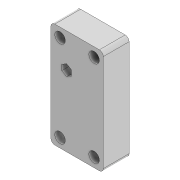
# Autodesk Inventor part: 10_Mountinplate_Mirrors_v2_Special_Combiner
Saved by Autodesk Inventor 2022 (Build 260153000, 153)
## iProperties
Created: 2022-05-18
Part Number: 10_Mountinplate_Mirrors_v2_Special_Combiner
Material: Generisch
Document SubType Name: Modeling
Designer: diederichbenedict
Density: 1 g/cm^3
Appearance: Vorgabe
Author: diederichbenedict
Autodesk Inventor part; units mm, degrees
ref_plane "YZ Plane" through (0, 0, 0) normal (1, 0, 0) x (0, 1, 0)
ref_plane "XZ Plane" through (0, 0, 0) normal (0, 1, 0) x (-1, 0, 0)
ref_plane "XY Plane" through (0, 0, 0) normal (0, 0, 1) x (1, 0, 0)
ref_plane "Arbeitsebene1" through (0.0075, -0.0423, 0) normal (0, 0, 1) x (1, 0, 0)
sketch "Skizze1" plane through (0.0075, -0.0423, 0) normal (0, 0, 1) x (1, 0, 0)
  line L0 (0.635, 25.527) -> (10.16, 25.527) projected
  line L1 (0.635, 25.527) -> (0.635, 0) projected
  line L2 (0.635, 0) -> (10.16, 0) projected
  line L3 (10.16, 0) -> (10.16, 25.527) projected
  line L4 (30.08, -27.3) -> (-3.92, -27.3)
  line L5 (-6.92, -24.3) -> (-6.92, 49.7)
  line L6 (-3.92, 52.7) -> (30.08, 52.7)
  line L7 (33.08, -27.3) -> (-6.92, 52.7) construction
  line L8 (-6.92, -27.3) -> (33.08, 52.7) construction
  arc A0 (30.08, -27.3) -> (33.08, -24.3) centre (30.08, -24.3) ccw
  arc A1 (-6.92, -24.3) -> (-3.92, -27.3) centre (-3.92, -24.3) ccw
  arc A2 (-3.92, 52.7) -> (-6.92, 49.7) centre (-3.92, 49.7) ccw
  arc A3 (33.08, 49.7) -> (30.08, 52.7) centre (30.08, 49.7) ccw
  circle A4 centre (5.08, 12.7) radius 2.3813
  line L9 (33.08, -24.3) -> (33.08, 49.7)
  line L10 (5.08, 12.7) -> (5.08, 26.7)
  circle A5 centre (5.08, 26.7) radius 2.3813
  point P0 (-0.0075, 0.0423)
  point P1 (13.08, 12.7)
  dimension "d1" = 80
  dimension "d2" = 3
  dimension "d7" = 0
  dimension "d8" = 8
  dimension "d37" = 14
  constraints: 14 end point, 8 point on circle, 7 tangent, 6 centre point, 6 point on line, 3 equal radius, 2 vertical, 1 horizontal, 1 midpoint, 1 parallel, 1 perpendicular, 2 other
  measures "d1" distance of L8.start L7.end
  measures "d2" radius of A0
  measures "d7" vertical distance of L10.start point (13.08, 12.7)
  measures "d8" distance of point (13.08, 12.7) L10.start
  measures "d37" distance of L10.start L10.end
ref_plane "Arbeitsebene2" through (291.5074, -13.3966, 8.6065) normal (0, 0, 1) x (0.898794, -0.4383711, 0)
extrude "Extrusion1" add sketch "Skizze1" along normal blind 18.412 contours L0 A5 L3 L2 L1 | L4 A1 L5 A2 L6 A3 L9 A0 | A4
sketch "Skizze3" plane through (0.0075, -0.0423, 0) normal (0, 0, -1) x (-1, 0, 0)
  arc A0 (-30.08, 52.7) -> (-33.08, 49.7) centre (-30.08, 49.7) ccw projected
  line L0 (-33.08, -24.3) -> (-33.08, 49.7) projected
  arc A1 (-33.08, -24.3) -> (-30.08, -27.3) centre (-30.08, -24.3) ccw projected
  line L1 (3.92, -27.3) -> (-30.08, -27.3) projected
  arc A2 (3.92, -27.3) -> (6.92, -24.3) centre (3.92, -24.3) ccw projected
  line L2 (6.92, 49.7) -> (6.92, -24.3) projected
  arc A3 (6.92, 49.7) -> (3.92, 52.7) centre (3.92, 49.7) ccw projected
  line L3 (-30.08, 52.7) -> (3.92, 52.7) projected
  line L4 (-26.08, 45.7) -> (-0.08, 45.7)
  line L5 (-0.08, 45.7) -> (-0.08, -20.3)
  line L6 (-0.08, -20.3) -> (-26.08, -20.3)
  line L7 (-26.08, -20.3) -> (-26.08, 45.7)
  point P0 (0.0075, 0.0423)
  dimension "d9" = 7
  constraints: 8 end point, 3 other
  measures "d9" distance between parallel lines of L0 L7
hole "Bohrung1" at (26.0875, 45.6577, 0) at (26.0875, -20.3423, 0) at (0.0875, -20.3423, 0) at (0.0875, 45.6577, 0) direction (0, 0, 1) diameter 8 end through all
sketch "Skizze4" plane through (-6.9125, -24.3423, 0) normal (-1, 0, 0) x (0, 0, 1)
  circle A0 centre (-6.731, 17.9923) radius 7.366 projected
  circle A1 centre (-6.731, 17.9923) radius 9.366
  circle A2 centre (-6.731, 56.05) radius 7.366
  circle A3 centre (-6.731, 56.05) radius 9.366
  line L0 (-6.731, 17.9923) -> (-6.731, 26.9923)
  circle A4 centre (-6.731, 26.9923) radius 9.366
  line L1 (-6.731, 56.05) -> (-6.731, 65.05)
  circle A5 centre (-6.731, 65.05) radius 9.366
  point P0 (0, 24.3423)
  dimension "d17" = 2
  dimension "d35" = 9
  dimension "d45" = 9
  constraints: 5 centre point, 4 end point, 2 vertical, 1 equal radius, 3 other
  measures "d17" radial gap between concentric circles of A0 A1
  measures "d35" distance of L0.start L0.end
  measures "d45" distance of L1.start L1.end
ref_plane "Arbeitsebene3" through (0, -11.176, -49.276) normal (-1, 0, 0) x (0, 0.0000004, 1)
extrude "Extrusion2" cut sketch "Skizze4" against normal up to surface (6.9125 mm away) contours A4 A0 | A0 A4 A1 | A1 A4 | A5 A2 | A2 A5 A3 | A3 A5 picked at (-6.731, 20.2469) picked at (0.3309, 22.9964) picked at (-6.731, 58.3046) picked at (0.3309, 61.0541)
sketch "Skizze5" plane through (0.0075, -0.0423, 0) normal (0, 0, -1) x (-1, 0, 0)
  line L0 (0.0075, -3.8204) -> (0.0075, 9.2051) projected
  line L1 (6.92, 34.2373) -> (6.92, 9.2051) projected
  arc A0 (6.92, 49.7) -> (3.92, 52.7) centre (3.92, 49.7) ccw projected
  line L2 (-30.08, 52.7) -> (3.92, 52.7) projected
  arc A1 (-30.08, 52.7) -> (-33.08, 49.7) centre (-30.08, 49.7) ccw projected
  line L3 (-33.08, -24.3) -> (-33.08, 49.7) projected
  arc A2 (-33.08, -24.3) -> (-30.08, -27.3) centre (-30.08, -24.3) ccw projected
  line L4 (3.92, -27.3) -> (-30.08, -27.3) projected
  arc A3 (3.92, -27.3) -> (6.92, -24.3) centre (3.92, -24.3) ccw projected
  line L5 (6.92, 49.7) -> (6.92, 47.2627) projected
  arc A4 (3.6021, 47.2627) -> (0.0075, 41.701) centre (-0.08, 45.7) ccw projected
  circle A5 centre (-26.08, -20.3) radius 4 projected
  circle A6 centre (-26.08, 45.7) radius 4 projected
  circle A7 centre (-0.08, -20.3) radius 4 projected
  line L6 (-0.6275, 29.1761) -> (-10.1525, 29.1761) projected
  line L7 (-0.6275, -2.2391) -> (-10.1525, -2.2391) projected
  line L8 (-10.1525, -2.2391) -> (-10.1525, 29.1761)
  line L9 (0.0075, 0.2051) -> (0.0075, -12.8204) projected
  line L10 (-10.3525, 29.3761) -> (-0.4275, 29.3761)
  line L11 (-0.4275, -2.4391) -> (-10.3525, -2.4391)
  line L12 (-12.6873, 36.83) -> (-19.1643, 36.83)
  line L13 (-12.6873, 17.399) -> (-12.6873, 4.5974)
  line L14 (-19.7993, 21.1275) -> (-19.7993, 26.543)
  line L15 (-22.9993, -3.011) -> (-22.9993, 36.83)
  line L16 (-22.9993, 36.83) -> (-12.6873, 36.83)
  line L17 (-12.4873, -3.011) -> (-12.4873, 37.03)
  line L18 (-12.4873, 37.03) -> (-23.1993, 37.03)
  line L19 (-26.1993, 37.03) -> (-23.1993, 37.03)
  line L20 (0, -0.127) -> (0, 25.4)
  line L21 (0, -0.127) -> (0, 25.4)
  line L22 (-0.4275, -2.4391) -> (0.0075, -2.4391)
  line L23 (0.2725, 29.3761) -> (-0.4275, 29.3761)
  line L24 (-10.3525, 6.561) -> (-10.3525, 38.361)
  line L25 (-5.08, 12.7) -> (-5.08, 21.7)
  circle A8 centre (-5.08, 21.7) radius 2.3815
  line L26 (-10.3525, 38.361) -> (-10.3525, 6.561)
  line L27 (-12.4873, -3.011) -> (-22.9993, -3.011)
  line L28 (-22.9993, -3.011) -> (-22.9993, 46.03)
  line L29 (-22.9993, 46.03) -> (-12.4873, 46.03)
  line L30 (-12.4873, 46.03) -> (-12.4873, -3.011)
  line L31 (6.92, -3.8204) -> (0.0075, -3.8204) projected
  line L32 (0.0075, 9.2051) -> (6.92, 9.2051) projected
  line L33 (0, 6.561) -> (-10.3525, 6.561)
  line L34 (-10.3525, 6.561) -> (-10.3525, 38.376)
  line L35 (-10.3525, 38.376) -> (0, 38.376)
  line L36 (0, 38.376) -> (0, 6.561)
  line L37 (0, 6.561) -> (0.0075, 6.561)
  line L38 (0.0075, 9.2051) -> (0.0075, -3.8204) projected
  line L39 (-22.9993, -3.011) -> (-26.1993, -3.011)
  line L40 (-26.1993, -3.011) -> (-26.1993, 46.03)
  line L41 (-26.1993, 46.03) -> (-22.9993, 46.03)
  line L42 (-22.9993, 46.03) -> (-22.9993, -3.011)
  line L43 (-10.3525, 38.376) -> (-12.4873, 38.376)
  line L44 (-12.4873, 38.376) -> (-12.4873, 6.561)
  line L45 (-12.4873, 6.561) -> (-10.3525, 6.561)
  line L46 (-10.3525, 6.561) -> (-10.3525, 38.376)
  line L47 (6.92, 34.2373) -> (0.0075, 34.2373) projected
  line L48 (0.0075, 34.2373) -> (0.0075, 41.701) projected
  line L49 (3.6021, 47.2627) -> (6.92, 47.2627) projected
  line L50 (6.92, -3.8204) -> (6.92, -24.3) projected
  line L51 (-12.4873, 38.376) -> (0.0075, 38.376)
  line L52 (0.0075, 38.376) -> (0.0075, 42.376)
  line L53 (0.0075, 42.376) -> (-12.4873, 42.376)
  line L54 (-12.4873, 42.376) -> (-12.4873, 38.376)
  point P0 (0.0075, 0.0423)
  point P1 (-22.9993, -3.011)
  point P2 (-22.9993, 43.1487)
  point P3 (-22.0936, 46.03)
  point P4 (-10.1525, 6.561)
  point P5 (-22.9993, 37.03)
  point P6 (0, 6.561)
  point P7 (0, 6.561)
  point P8 (-26.1993, 41.7018)
  point P9 (-2.3051, 42.376)
  point P10 (0.0075, 38.376)
  point P11 (0, 38.376)
  dimension "d27" = 3
  dimension "d28" = 0.7
  dimension "d30" = 31.8
  dimension "d31" = 9
  dimension "d32" = 4.763
  dimension "d33" = 49.041
  dimension "d34" = 10.512
  dimension "d36" = 31.815
  dimension "d46" = 4
  constraints: 78 end point, 11 parallel, 8 horizontal, 5 perpendicular, 5 point on line, 5 vertical, 1 centre point, 1 coincident, 8 other
  measures "d27" distance of L19.start L19.end
  measures "d28" distance of L23.end L23.start
  measures "d30" distance of L24.start L24.end
  measures "d31" distance of L25.start L25.end
  measures "d32" diameter of A8
  measures "d33" distance of L15.start L28.end
  measures "d34" distance of L28.end L29.end
  measures "d36" distance of L33.end L34.end
  measures "d46" distance of L52.end L51.end
ref_plane "Arbeitsebene4" through (-0.1034, 27.5049, -1.27) normal (0, 0.0000004, 1) x (1, 0, 0)
extrude "Extrusion3" add sketch "Skizze5" along normal up to surface (1.27 mm away) contours L31 L50 A3 L4 A2 L3 A1 L2 A0 L5 L49 A4 L53 L30 L29 A6 L40 L39 L27 L17 L45 L33 L37 L0 | L37 L20 L36 L51 L48 L47 L1 L32 L0
sketch "Sketch6" plane through (0.0075, -0.0423, 18.412) normal (0, 0, 1) x (1, 0, 0)
  circle A0 centre (5.08, 12.7) radius 2.3813 projected
  line L0 (8.8085, 14.7861) -> (8.7509, 10.5141)
  line L1 (8.7509, 10.5141) -> (5.0224, 8.428)
  line L2 (5.0224, 8.428) -> (1.3515, 10.6139)
  line L3 (1.3515, 10.6139) -> (1.4091, 14.8859)
  line L4 (1.4091, 14.8859) -> (5.1376, 16.972)
  line L5 (5.1376, 16.972) -> (8.8085, 14.7861)
  circle A1 centre (5.08, 26.7) radius 2.3813 projected
  line L6 (5.08, 12.7) -> (5.08, 26.7)
  line L7 (5.08, 22.4276) -> (1.38, 24.5638)
  line L8 (1.38, 24.5638) -> (1.38, 28.8362)
  line L9 (1.38, 28.8362) -> (5.08, 30.9724)
  line L10 (5.08, 30.9724) -> (8.78, 28.8362)
  line L11 (8.78, 28.8362) -> (8.78, 24.5638)
  line L12 (8.78, 24.5638) -> (5.08, 22.4276)
  point P0 (-0.0075, 0.0423)
  dimension "d23" = 3.7
  dimension "d38" = 14
  dimension "d47" = 3.7
  constraints: 26 end point, 2 coincident, 1 point on line, 1 vertical, 26 other
  measures "d23" distance from line of L4 A0.centre
  measures "d38" distance of L6.start L6.end
  measures "d47" distance from line of L6.end L12
extrude "Extrusion4" cut sketch "Sketch6" against normal blind 10 contours L7 L8 L9 L10 L11 L12
sketch "Sketch7" plane through (30.0875, 52.6577, -1.27) normal (0, -0.0000004, -1) x (-1, 0, 0)
  circle A0 centre (30, -73) radius 4 projected
  circle A1 centre (30, -73) radius 6.5
  circle A2 centre (4, -73) radius 4 projected
  circle A3 centre (4, -73) radius 6.5
  circle A4 centre (30, -7) radius 4 projected
  circle A5 centre (30, -7) radius 6.5
  circle A6 centre (4, -7) radius 4 projected
  circle A7 centre (4, -7) radius 6.5
  point P0 (30.0875, -52.6577)
  dimension "d39" = 13
  dimension "d40" = 13
  dimension "d41" = 13
  dimension "d42" = 13
  constraints: 4 centre point, 4 coincident
  measures "d39" diameter of A1
  measures "d40" diameter of A3
  measures "d41" diameter of A5
  measures "d42" diameter of A7
extrude "Extrusion5" cut sketch "Sketch7" against normal blind 8 contours A0 | A1 | A3 | A5 | A7
fillet "Fillet1" radius 0.5 7 edges at (12.4948, 1.7327, -1.27) (6.2511, 6.5187, -1.27) (0.0075, 22.4262, -1.27) (12.4948, 44.1607, -1.27) (16.0453, 45.9877, -1.27) (26.2068, 18.0527, -1.27) (19.3508, -3.0533, -1.27)
